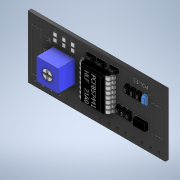
# Autodesk Inventor part: Part2_I2C
Saved by Autodesk Inventor 2021 (Build 250183000, 183)
## iProperties
Created: 2022-06-25
Part Number: Part2_I2C
Material: Generic
Document SubType Name: Modeling
Designer: Sam14
Density: 1 g/cm^3
Appearance: Chrome - Polished
Author: Sam14
Autodesk Inventor part; units mm, degrees
(part 1 of 3)
ref_plane "YZ Plane" through (0, 0, 0) normal (1, 0, 0) x (0, 1, 0)
ref_plane "XZ Plane" through (0, 0, 0) normal (0, 1, 0) x (-1, 0, 0)
sketch "Sketch1" plane through (0, 0, 0) normal (0, 0, 1) x (1, 0, 0)
  line L0 (0, 0) -> (38.1, 0)
  line L1 (0.325, -0.325) -> (0.325, 0.325)
  line L2 (0.325, 0.325) -> (-0.325, 0.325)
  line L3 (-0.325, 0.325) -> (-0.325, -0.325)
  line L4 (-0.325, -0.325) -> (0.325, -0.325)
  line L5 (0.325, -0.325) -> (-0.325, 0.325) construction
  line L6 (0.325, 0.325) -> (-0.325, -0.325) construction
  line L7 (38.425, -0.325) -> (37.775, -0.325)
  line L8 (37.775, -0.325) -> (37.775, 0.325)
  line L9 (37.775, 0.325) -> (38.425, 0.325)
  line L10 (38.425, 0.325) -> (38.425, -0.325)
  line L11 (38.425, -0.325) -> (37.775, 0.325) construction
  line L12 (37.775, -0.325) -> (38.425, 0.325) construction
  line L13 (0, 0) -> (2.54, 0)
  line L14 (2.54, 0) -> (5.08, 0)
  line L15 (5.08, 0) -> (7.62, 0)
  line L16 (7.62, 0) -> (10.16, 0)
  line L17 (10.16, 0) -> (12.7, 0)
  line L18 (12.7, 0) -> (15.24, 0)
  line L19 (15.24, 0) -> (17.78, 0)
  line L20 (17.78, 0) -> (20.32, 0)
  line L21 (20.32, 0) -> (22.86, 0)
  line L22 (22.86, 0) -> (25.4, 0)
  line L23 (25.4, 0) -> (27.94, 0)
  line L24 (27.94, 0) -> (30.48, 0)
  line L25 (30.48, 0) -> (33.02, 0)
  line L26 (33.02, 0) -> (35.56, 0)
  line L27 (35.56, 0) -> (38.1, 0)
  line L28 (-0.325, 0.325) -> (0.325, -0.325)
  line L29 (0.325, 0.325) -> (-0.325, -0.325)
  line L30 (2.865, -0.325) -> (2.865, 0.325)
  line L31 (2.865, 0.325) -> (2.215, 0.325)
  line L32 (2.215, 0.325) -> (2.215, -0.325)
  line L33 (2.215, -0.325) -> (2.865, -0.325)
  line L34 (2.865, -0.325) -> (2.215, 0.325) construction
  line L35 (2.865, 0.325) -> (2.215, -0.325) construction
  line L36 (5.405, -0.325) -> (5.405, 0.325)
  line L37 (5.405, 0.325) -> (4.755, 0.325)
  line L38 (4.755, 0.325) -> (4.755, -0.325)
  line L39 (4.755, -0.325) -> (5.405, -0.325)
  line L40 (5.405, -0.325) -> (4.755, 0.325) construction
  line L41 (5.405, 0.325) -> (4.755, -0.325) construction
  line L42 (7.945, -0.325) -> (7.945, 0.325)
  line L43 (7.945, 0.325) -> (7.295, 0.325)
  line L44 (7.295, 0.325) -> (7.295, -0.325)
  line L45 (7.295, -0.325) -> (7.945, -0.325)
  line L46 (7.945, -0.325) -> (7.295, 0.325) construction
  line L47 (7.945, 0.325) -> (7.295, -0.325) construction
  line L48 (10.485, -0.325) -> (10.485, 0.325)
  line L49 (10.485, 0.325) -> (9.835, 0.325)
  line L50 (9.835, 0.325) -> (9.835, -0.325)
  line L51 (9.835, -0.325) -> (10.485, -0.325)
  line L52 (10.485, -0.325) -> (9.835, 0.325) construction
  line L53 (10.485, 0.325) -> (9.835, -0.325) construction
  line L54 (13.025, -0.325) -> (13.025, 0.325)
  line L55 (13.025, 0.325) -> (12.375, 0.325)
  line L56 (12.375, 0.325) -> (12.375, -0.325)
  line L57 (12.375, -0.325) -> (13.025, -0.325)
  line L58 (13.025, -0.325) -> (12.375, 0.325) construction
  line L59 (13.025, 0.325) -> (12.375, -0.325) construction
  line L60 (15.565, -0.325) -> (15.565, 0.325)
  line L61 (15.565, 0.325) -> (14.915, 0.325)
  line L62 (14.915, 0.325) -> (14.915, -0.325)
  line L63 (14.915, -0.325) -> (15.565, -0.325)
  line L64 (15.565, -0.325) -> (14.915, 0.325) construction
  line L65 (15.565, 0.325) -> (14.915, -0.325) construction
  line L66 (18.105, -0.325) -> (18.105, 0.325)
  line L67 (18.105, 0.325) -> (17.455, 0.325)
  line L68 (17.455, 0.325) -> (17.455, -0.325)
  line L69 (17.455, -0.325) -> (18.105, -0.325)
  line L70 (18.105, -0.325) -> (17.455, 0.325) construction
  line L71 (18.105, 0.325) -> (17.455, -0.325) construction
  line L72 (20.645, -0.325) -> (20.645, 0.325)
  line L73 (20.645, 0.325) -> (19.995, 0.325)
  line L74 (19.995, 0.325) -> (19.995, -0.325)
  line L75 (19.995, -0.325) -> (20.645, -0.325)
  line L76 (20.645, -0.325) -> (19.995, 0.325) construction
  line L77 (20.645, 0.325) -> (19.995, -0.325) construction
  line L78 (23.185, -0.325) -> (23.185, 0.325)
  line L79 (23.185, 0.325) -> (22.535, 0.325)
  line L80 (22.535, 0.325) -> (22.535, -0.325)
  line L81 (22.535, -0.325) -> (23.185, -0.325)
  line L82 (23.185, -0.325) -> (22.535, 0.325) construction
  line L83 (23.185, 0.325) -> (22.535, -0.325) construction
  line L84 (25.725, -0.325) -> (25.725, 0.325)
  line L85 (25.725, 0.325) -> (25.075, 0.325)
  line L86 (25.075, 0.325) -> (25.075, -0.325)
  line L87 (25.075, -0.325) -> (25.725, -0.325)
  line L88 (25.725, -0.325) -> (25.075, 0.325) construction
  line L89 (25.725, 0.325) -> (25.075, -0.325) construction
  line L90 (28.265, -0.325) -> (28.265, 0.325)
  line L91 (28.265, 0.325) -> (27.615, 0.325)
  line L92 (27.615, 0.325) -> (27.615, -0.325)
  line L93 (27.615, -0.325) -> (28.265, -0.325)
  line L94 (28.265, -0.325) -> (27.615, 0.325) construction
  line L95 (28.265, 0.325) -> (27.615, -0.325) construction
  line L96 (30.805, -0.325) -> (30.805, 0.325)
  line L97 (30.805, 0.325) -> (30.155, 0.325)
  line L98 (30.155, 0.325) -> (30.155, -0.325)
  line L99 (30.155, -0.325) -> (30.805, -0.325)
  line L100 (30.805, -0.325) -> (30.155, 0.325) construction
  line L101 (30.805, 0.325) -> (30.155, -0.325) construction
  line L102 (33.345, -0.325) -> (33.345, 0.325)
  line L103 (33.345, 0.325) -> (32.695, 0.325)
  line L104 (32.695, 0.325) -> (32.695, -0.325)
  line L105 (32.695, -0.325) -> (33.345, -0.325)
  line L106 (33.345, -0.325) -> (32.695, 0.325) construction
  line L107 (33.345, 0.325) -> (32.695, -0.325) construction
  line L108 (35.885, -0.325) -> (35.885, 0.325)
  line L109 (35.885, 0.325) -> (35.235, 0.325)
  line L110 (35.235, 0.325) -> (35.235, -0.325)
  line L111 (35.235, -0.325) -> (35.885, -0.325)
  line L112 (35.885, -0.325) -> (35.235, 0.325) construction
  line L113 (35.885, 0.325) -> (35.235, -0.325) construction
  line L114 (0, 0) -> (-1.95, 0)
  line L115 (38.1, 0) -> (40.05, 0)
  line L116 (40.05, 0) -> (40.05, -1.5)
  line L117 (-1.95, 0) -> (-1.95, -1.5)
  line L118 (-1.95, -1.5) -> (40.05, -1.5)
  line L119 (40.05, -1.5) -> (40.05, 17.5)
  line L120 (-1.95, -1.5) -> (-1.95, 17.5)
  line L121 (-1.95, 17.5) -> (40.05, 17.5)
  dimension "d53" = 38.1
  dimension "d54" = 0.65
  dimension "d55" = 0.65
  dimension "d56" = 0.65
  dimension "d57" = 0.65
  dimension "d58" = 2.54
  dimension "d59" = 2.54
  dimension "d60" = 2.54
  dimension "d61" = 2.54
  dimension "d62" = 2.54
  dimension "d63" = 2.54
  dimension "d64" = 2.54
  dimension "d65" = 2.54
  dimension "d66" = 2.54
  dimension "d67" = 2.54
  dimension "d68" = 2.54
  dimension "d69" = 2.54
  dimension "d70" = 2.54
  dimension "d71" = 2.54
  dimension "d72" = 0.65
  dimension "d73" = 0.65
  dimension "d74" = 0.65
  dimension "d75" = 0.65
  dimension "d76" = 0.65
  dimension "d77" = 0.65
  dimension "d78" = 0.65
  dimension "d79" = 0.65
  dimension "d80" = 0.65
  dimension "d81" = 0.65
  dimension "d82" = 0.65
  dimension "d83" = 0.65
  dimension "d84" = 0.65
  dimension "d85" = 0.65
  dimension "d86" = 0.65
  dimension "d87" = 0.65
  dimension "d88" = 0.65
  dimension "d89" = 0.65
  dimension "d90" = 0.65
  dimension "d91" = 0.65
  dimension "d92" = 0.65
  dimension "d93" = 0.65
  dimension "d94" = 0.65
  dimension "d95" = 0.65
  dimension "d96" = 0.65
  dimension "d97" = 0.65
  dimension "d98" = 0.65
  dimension "d99" = 0.65
  dimension "d100" = 1.95
  dimension "d101" = 1.95
  dimension "d102" = 1.5
  dimension "d103" = 1.5
  dimension "d104" = 19
  dimension "d105" = 19
  constraints: 242 end point, 32 parallel, 18 vertical, 16 perpendicular, 4 midpoint, 3 horizontal, 1 point on line, 17 other
  measures "d53" distance of L13.start L27.end
  measures "d54" distance of L1.start L1.end
  measures "d55" distance of L2.end L1.end
  measures "d56" distance of L7.start L7.end
  measures "d57" distance of L7.end L8.end
  measures "d58" distance of L13.start L13.end
  measures "d59" distance of L13.end L14.end
  measures "d60" distance of L14.end L15.end
  measures "d61" distance of L15.end L16.end
  measures "d62" distance of L16.end L17.end
  measures "d63" distance of L17.end L18.end
  measures "d64" distance of L18.end L19.end
  measures "d65" distance of L19.end L20.end
  measures "d66" distance of L20.end L21.end
  measures "d67" distance of L21.end L22.end
  measures "d68" distance of L22.end L23.end
  measures "d69" distance of L23.end L24.end
  measures "d70" distance of L24.end L25.end
  measures "d71" distance of L25.end L26.end
  measures "d72" distance of L34.start L31.start
  measures "d73" distance of L31.end L31.start
  measures "d74" distance of L40.start L37.start
  measures "d75" distance of L37.end L37.start
  measures "d76" distance of L46.start L43.start
  measures "d77" distance of L43.end L43.start
  measures "d78" distance of L52.start L49.start
  measures "d79" distance of L49.end L49.start
  measures "d80" distance of L58.start L55.start
  measures "d81" distance of L55.end L55.start
  measures "d82" distance of L64.start L61.start
  measures "d83" distance of L61.end L61.start
  measures "d84" distance of L70.start L67.start
  measures "d85" distance of L67.end L67.start
  measures "d86" distance of L76.start L73.start
  measures "d87" distance of L73.end L73.start
  measures "d88" distance of L82.start L79.start
  measures "d89" distance of L79.end L79.start
  measures "d90" distance of L88.start L85.start
  measures "d91" distance of L85.end L85.start
  measures "d92" distance of L94.start L91.start
  measures "d93" distance of L91.end L91.start
  measures "d94" distance of L100.start L97.start
  measures "d95" distance of L97.end L97.start
  measures "d96" distance of L106.start L103.start
  measures "d97" distance of L103.end L103.start
  measures "d98" distance of L112.start L109.start
  measures "d99" distance of L109.end L109.start
  measures "d100" distance of L13.start L114.end
  measures "d101" distance of L27.end L115.end
  measures "d102" distance of L115.end L116.end
  measures "d103" distance of L114.end L117.end
  measures "d104" distance of L116.end L119.end
  measures "d105" distance of L117.end L120.end
extrude "Extrusion1" add sketch "Sketch1" along normal blind 1 contours L1 L2 L3 L114 L120 L121 L119 L115 L10 L9 L8 L0 L108 L109 L110 L102 L103 L104 L96 L97 L98 L90 L91 L92 L84 L85 L86 L78 L79 L80 L72 L73 L74 L66 L67 L68 L60 L61 L62 L54 L55 L56 L48 L49 L50 L42 L43 L44 L36 L37 L38 L30 L31 L32 | L0 L32 L33 L30 L38 L39 L36 L44 L45 L42 L50 L51 L48 L56 L57 L54 L62 L63 L60 L68 L69 L66 L74 L75 L72 L80 L81 L78 L86 L87 L84 L92 L93 L90 L98 L99 L96 L104 L105 L102 L110 L111 L108 L8 L7 L10 L115 L116 L118 L117 L114 L3 L4 L1
sketch "Sketch2" plane through (0, 0, 1) normal (0, 0, 1) x (1, 0, 0)
  line L0 (5.55, 12) -> (12.55, 12)
  line L1 (12.55, 12) -> (12.55, 5)
  line L2 (12.55, 5) -> (5.55, 5)
  line L3 (5.55, 5) -> (5.55, 12)
  line L4 (5.65, 5.1) -> (12.45, 5.1)
  line L5 (12.45, 5.1) -> (12.45, 11.9)
  line L6 (12.45, 11.9) -> (5.65, 11.9)
  line L7 (5.65, 11.9) -> (5.65, 5.1)
  line L8 (-0.95, 14.5) -> (-0.95, 1.5)
  line L9 (2.05, 14.5) -> (2.05, 1.5)
  line L10 (-0.95, 14.5) -> (2.05, 14.5)
  line L11 (-0.95, 1.5) -> (2.05, 1.5)
  line L12 (1.95, 14.4) -> (1.95, 1.6)
  line L13 (1.95, 1.6) -> (-0.85, 1.6)
  line L14 (-0.85, 1.6) -> (-0.85, 14.4)
  line L15 (-0.85, 14.4) -> (1.95, 14.4)
  line L16 (40.05, -1.5) -> (40.05, 17.5) projected
  line L17 (36.05, 4) -> (36.05, 12)
  line L18 (36.05, 12) -> (39.05, 12)
  line L19 (39.05, 4) -> (36.05, 4)
  line L20 (39.05, 12) -> (39.05, 4)
  line L21 (39.15, 12.1) -> (35.95, 12.1)
  line L22 (35.95, 12.1) -> (35.95, 3.9)
  line L23 (35.95, 3.9) -> (39.15, 3.9)
  line L24 (39.15, 3.9) -> (39.15, 12.1)
  line L25 (34.95, 3.9) -> (34.95, 6.4)
  line L26 (34.95, 6.4) -> (30.95, 6.4)
  line L27 (30.95, 6.4) -> (30.95, 3.9)
  line L28 (30.95, 3.9) -> (34.95, 3.9)
  line L29 (34.85, 4) -> (34.85, 6.3)
  line L30 (34.85, 6.3) -> (31.05, 6.3)
  line L31 (31.05, 6.3) -> (31.05, 4)
  line L32 (31.05, 4) -> (34.85, 4)
  line L33 (29.95, 3.9) -> (29.95, 6.9)
  line L34 (29.95, 6.9) -> (28.45, 6.9)
  line L35 (28.45, 6.9) -> (28.45, 3.9)
  line L36 (28.45, 3.9) -> (29.95, 3.9)
  line L37 (39.15, 3.9) -> (40.05, 3.9)
  line L38 (29.85, 6.8) -> (29.85, 4)
  line L39 (29.85, 4) -> (28.55, 4)
  line L40 (28.55, 4) -> (28.55, 6.8)
  line L41 (28.55, 6.8) -> (29.85, 6.8)
  line L42 (28.45, 3.9) -> (28.45, 6.9)
  line L43 (28.45, 6.9) -> (26.95, 6.9)
  line L44 (26.95, 6.9) -> (26.95, 3.9)
  line L45 (26.95, 3.9) -> (28.45, 3.9)
  line L46 (28.35, 6.8) -> (28.35, 4)
  line L47 (28.35, 4) -> (27.05, 4)
  line L48 (27.05, 4) -> (27.05, 6.8)
  line L49 (27.05, 6.8) -> (28.35, 6.8)
  line L50 (26.95, 3.9) -> (26.95, 6.9)
  line L51 (26.95, 6.9) -> (25.45, 6.9)
  line L52 (25.45, 6.9) -> (25.45, 3.9)
  line L53 (25.45, 3.9) -> (26.95, 3.9)
  line L54 (26.85, 6.8) -> (26.85, 4)
  line L55 (26.85, 4) -> (25.55, 4)
  line L56 (25.55, 4) -> (25.55, 6.8)
  line L57 (25.55, 6.8) -> (26.85, 6.8)
  line L58 (34.95, 10.5872) -> (34.95, 13.5872)
  line L59 (34.95, 13.5872) -> (33.45, 13.5872)
  line L60 (33.45, 13.5872) -> (33.45, 10.5872)
  line L61 (33.45, 10.5872) -> (34.95, 10.5872)
  line L62 (34.85, 13.4872) -> (34.85, 10.6872)
  line L63 (34.85, 10.6872) -> (33.55, 10.6872)
  line L64 (33.55, 10.6872) -> (33.55, 13.4872)
  line L65 (33.55, 13.4872) -> (34.85, 13.4872)
  line L66 (33.1382, 10.6872) -> (33.1382, 13.6872)
  line L67 (33.1382, 13.6872) -> (31.6382, 13.6872)
  line L68 (31.6382, 13.6872) -> (31.6382, 10.6872)
  line L69 (31.6382, 10.6872) -> (33.1382, 10.6872)
  line L70 (33.0382, 13.5872) -> (33.0382, 10.7872)
  line L71 (33.0382, 10.7872) -> (31.7382, 10.7872)
  line L72 (31.7382, 10.7872) -> (31.7382, 13.5872)
  line L73 (31.7382, 13.5872) -> (33.0382, 13.5872)
  line L74 (31.3887, 10.6872) -> (31.3887, 13.6872)
  line L75 (31.3887, 13.6872) -> (29.8887, 13.6872)
  line L76 (29.8887, 13.6872) -> (29.8887, 10.6872)
  line L77 (29.8887, 10.6872) -> (31.3887, 10.6872)
  line L78 (31.2887, 13.5872) -> (31.2887, 10.7872)
  line L79 (31.2887, 10.7872) -> (29.9887, 10.7872)
  line L80 (29.9887, 10.7872) -> (29.9887, 13.5872)
  line L81 (29.9887, 13.5872) -> (31.2887, 13.5872)
  line L82 (29.5585, 10.6872) -> (29.5585, 13.6872)
  line L83 (29.5585, 13.6872) -> (28.0585, 13.6872)
  line L84 (28.0585, 13.6872) -> (28.0585, 10.6872)
  line L85 (28.0585, 10.6872) -> (29.5585, 10.6872)
  line L86 (29.4585, 13.5872) -> (29.4585, 10.7872)
  line L87 (29.4585, 10.7872) -> (28.1585, 10.7872)
  line L88 (28.1585, 10.7872) -> (28.1585, 13.5872)
  line L89 (28.1585, 13.5872) -> (29.4585, 13.5872)
  line L90 (7.1408, 13.077) -> (7.1408, 16.077)
  line L91 (7.1408, 16.077) -> (5.6408, 16.077)
  line L92 (5.6408, 16.077) -> (5.6408, 13.077)
  line L93 (5.6408, 13.077) -> (7.1408, 13.077)
  line L94 (7.0408, 15.977) -> (7.0408, 13.177)
  line L95 (7.0408, 13.177) -> (5.7408, 13.177)
  line L96 (5.7408, 13.177) -> (5.7408, 15.977)
  line L97 (5.7408, 15.977) -> (7.0408, 15.977)
  line L98 (9.8434, 13.0715) -> (9.8434, 16.0715)
  line L99 (9.8434, 16.0715) -> (8.3434, 16.0715)
  line L100 (8.3434, 16.0715) -> (8.3434, 13.0715)
  line L101 (8.3434, 13.0715) -> (9.8434, 13.0715)
  line L102 (9.7434, 15.9715) -> (9.7434, 13.1715)
  line L103 (9.7434, 13.1715) -> (8.4434, 13.1715)
  line L104 (8.4434, 13.1715) -> (8.4434, 15.9715)
  line L105 (8.4434, 15.9715) -> (9.7434, 15.9715)
  line L106 (12.545, 13.0887) -> (12.545, 16.0887)
  line L107 (12.545, 16.0887) -> (11.045, 16.0887)
  line L108 (11.045, 16.0887) -> (11.045, 13.0887)
  line L109 (11.045, 13.0887) -> (12.545, 13.0887)
  line L110 (12.445, 15.9887) -> (12.445, 13.1887)
  line L111 (12.445, 13.1887) -> (11.145, 13.1887)
  line L112 (11.145, 13.1887) -> (11.145, 15.9887)
  line L113 (11.145, 15.9887) -> (12.445, 15.9887)
  line L114 (-1.95, 17.5) -> (-1.95, -1.5) projected
  line L115 (-1.95, 17.5) -> (16.05, 17.5)
  line L116 (40.05, 17.5) -> (-1.95, 17.5) projected
  line L117 (16.05, 14) -> (23.45, 14)
  line L118 (23.45, 14) -> (23.45, 3.5)
  line L119 (23.45, 3.5) -> (16.05, 3.5)
  line L120 (16.05, 3.5) -> (16.05, 14)
  line L121 (15.95, 14.1) -> (23.55, 14.1)
  line L122 (23.55, 14.1) -> (23.55, 3.4)
  line L123 (23.55, 3.4) -> (15.95, 3.4)
  line L124 (15.95, 3.4) -> (15.95, 14.1)
  line L125 (19.0957, 15.9376) -> (16.0957, 15.9376)
  line L126 (16.1957, 15.8376) -> (18.9957, 15.8376)
  line L127 (18.9957, 15.8376) -> (18.9957, 14.5376)
  line L128 (19.0957, 14.4376) -> (19.0957, 15.9376)
  line L129 (18.9957, 14.5376) -> (16.1957, 14.5376)
  line L130 (16.1957, 14.5376) -> (16.1957, 15.8376)
  line L131 (16.0957, 14.4376) -> (19.0957, 14.4376)
  line L132 (16.0957, 15.9376) -> (16.0957, 14.4376)
  line L133 (22.1559, 15.8398) -> (22.1559, 14.5398)
  line L134 (19.2559, 15.9398) -> (19.2559, 14.4398)
  line L135 (19.2559, 14.4398) -> (22.2559, 14.4398)
  line L136 (22.2559, 14.4398) -> (22.2559, 15.9398)
  line L137 (19.3559, 14.5398) -> (19.3559, 15.8398)
  line L138 (19.3559, 15.8398) -> (22.1559, 15.8398)
  line L139 (22.1559, 14.5398) -> (19.3559, 14.5398)
  line L140 (22.2559, 15.9398) -> (19.2559, 15.9398)
  line L141 (26.0246, 15.977) -> (26.0246, 14.677)
  line L142 (23.1246, 16.077) -> (23.1246, 14.577)
  line L143 (23.1246, 14.577) -> (26.1246, 14.577)
  line L144 (26.1246, 14.577) -> (26.1246, 16.077)
  line L145 (23.2246, 14.677) -> (23.2246, 15.977)
  line L146 (23.2246, 15.977) -> (26.0246, 15.977)
  line L147 (26.0246, 14.677) -> (23.2246, 14.677)
  line L148 (26.1246, 16.077) -> (23.1246, 16.077)
  point P0 (0, 0)
  dimension "d111" = 7
  dimension "d112" = 0.1
  dimension "d114" = 3
  dimension "d117" = 0.1
  dimension "d121" = 0.1
  dimension "d123" = 2.5
  dimension "d124" = 4
  dimension "d125" = 0.1
  dimension "d126" = 1
  dimension "d127" = 3
  dimension "d128" = 1.5
  dimension "d129" = 0.9
  dimension "d131" = 0.1
  dimension "d132" = 3
  dimension "d133" = 1.5
  dimension "d134" = 0.1
  dimension "d135" = 3
  dimension "d136" = 1.5
  dimension "d137" = 0.1
  dimension "d138" = 3
  dimension "d139" = 1.5
  dimension "d140" = 0.1
  dimension "d141" = 3
  dimension "d142" = 1.5
  dimension "d143" = 0.1
  dimension "d144" = 3
  dimension "d145" = 1.5
  dimension "d146" = 0.1
  dimension "d147" = 3
  dimension "d148" = 1.5
  dimension "d149" = 0.1
  dimension "d150" = 3
  dimension "d151" = 1.5
  dimension "d152" = 0.1
  dimension "d153" = 3
  dimension "d154" = 1.5
  dimension "d155" = 0.1
  dimension "d156" = 3
  dimension "d157" = 1.5
  dimension "d158" = 0.1
  dimension "d159" = 18
  dimension "d160" = 3.5
  dimension "d161" = 7.4
  dimension "d162" = 10.5
  dimension "d163" = 0.1
  dimension "d164" = 3
  dimension "d165" = 1.5
  dimension "d166" = 0.1
  dimension "d167" = 3
  dimension "d168" = 1.5
  dimension "d169" = 0.1
  dimension "d170" = 3
  dimension "d171" = 1.5
  dimension "d172" = 0.1
  constraints: 292 end point, 100 perpendicular, 3 point on line, 2 parallel, 1 horizontal, 1 vertical, 54 other
  measures "d111" distance of L0.end L1.end
  measures "d112" distance between parallel lines of L2 L4
  measures "d114" distance between parallel lines of L8 L9
  measures "d117" distance between parallel lines of L10 L15
  measures "d121" distance between parallel lines of L18 L21
  measures "d123" distance of L25.start L25.end
  measures "d124" distance of L25.end L26.end
  measures "d125" distance between parallel lines of L28 L32
  measures "d126" distance of L27.end L33.start
  measures "d127" distance of L33.start L33.end
  measures "d128" distance of L33.end L34.end
  measures "d129" distance of L23.end L37.end
  measures "d131" distance between parallel lines of L33 L38
  measures "d132" distance of L42.start L43.start
  measures "d133" distance of L43.start L44.start
  measures "d134" distance between parallel lines of L42 L46
  measures "d135" distance of L50.start L51.start
  measures "d136" distance of L51.start L52.start
  measures "d137" distance between parallel lines of L50 L54
  measures "d138" distance of L58.start L59.start
  measures "d139" distance of L59.start L60.start
  measures "d140" distance between parallel lines of L58 L62
  measures "d141" distance of L66.start L67.start
  measures "d142" distance of L67.start L68.start
  measures "d143" distance between parallel lines of L66 L70
  measures "d144" distance of L74.start L75.start
  measures "d145" distance of L75.start L76.start
  measures "d146" distance between parallel lines of L74 L78
  measures "d147" distance of L82.start L83.start
  measures "d148" distance of L83.start L84.start
  measures "d149" distance between parallel lines of L82 L86
  measures "d150" distance of L90.start L91.start
  measures "d151" distance of L91.start L92.start
  measures "d152" distance between parallel lines of L90 L94
  measures "d153" distance of L98.start L99.start
  measures "d154" distance of L99.start L100.start
  measures "d155" distance between parallel lines of L98 L102
  measures "d156" distance of L106.start L107.start
  measures "d157" distance of L107.start L108.start
  measures "d158" distance between parallel lines of L106 L110
  measures "d159" distance of L114.start L115.end
  measures "d160" distance of L115.end L117.start
  measures "d161" distance of L117.start L117.end
  measures "d162" distance of L117.end L118.end
  measures "d163" distance between parallel lines of L120 L124
  measures "d164" distance of L132.end L131.end
  measures "d165" distance of L131.end L128.end
  measures "d166" distance between parallel lines of L131 L129
  measures "d167" distance of L134.end L136.start
  measures "d168" distance of L136.start L140.start
  measures "d169" distance between parallel lines of L135 L139
  measures "d170" distance of L142.end L144.start
  measures "d171" distance of L144.start L148.start
  measures "d172" distance between parallel lines of L143 L147
extrude "Extrusion2" add sketch "Sketch2" along normal blind 0.1
sketch "Sketch4" plane through (0, 0, 1) normal (0, 0, 1) x (1, 0, 0)
  line L0 (5.65, 5.1) -> (12.45, 5.1) projected
  line L1 (12.45, 5.1) -> (12.45, 11.9) projected
  line L2 (12.45, 11.9) -> (5.65, 11.9) projected
  line L3 (5.65, 11.9) -> (5.65, 5.1) projected
  line L4 (5.75, 11.8) -> (12.35, 11.8)
  line L5 (12.35, 11.8) -> (12.35, 5.2)
  line L6 (12.35, 5.2) -> (5.75, 5.2)
  line L7 (5.75, 5.2) -> (5.75, 11.8)
  point P0 (0, 0)
  dimension "d175" = 0.1
  constraints: 8 end point, 3 other
  measures "d175" distance between parallel lines of L2 L4
extrude "Extrusion3" add sketch "Sketch4" along normal blind 5.1 contours L4 L5 L6 L7
sketch "Sketch5" plane through (0, 0, 6.1) normal (0, 0, 1) x (1, 0, 0)
  line L0 (5.75, 5.2) -> (12.35, 5.2) projected
  line L1 (12.35, 5.2) -> (12.35, 11.8) projected
  line L2 (12.35, 11.8) -> (5.75, 11.8) projected
  line L3 (5.75, 11.8) -> (5.75, 5.2) projected
  line L4 (5.75, 11.8) -> (12.35, 5.2)
  line L5 (5.75, 5.2) -> (12.35, 11.8)
  circle A0 centre (9.05, 8.5) radius 1.5
  point P0 (0, 0)
  dimension "d178" = 3
  constraints: 4 end point, 1 centre point, 1 midpoint, 1 perpendicular
  measures "d178" diameter of A0
extrude "Extrusion4" cut sketch "Sketch5" against normal blind 1 contours A0 L4 L5 | L5 L4 A0 | L4 L5 A0 | A0 L5 L4
sketch "Sketch6" plane through (0, 0, 6.1) normal (0, 0, 1) x (1, 0, 0)
  circle A0 centre (9.05, 8.5) radius 1.5 projected
  circle A1 centre (9.05, 8.5) radius 1.75
  circle A2 centre (9.05, 8.5) radius 1.85
  point P0 (0, 0)
  dimension "d181" = 3.5
  dimension "d182" = 3.7
  constraints: 2 centre point, 2 coincident
  measures "d181" diameter of A1
  measures "d182" diameter of A2
extrude "Extrusion5" cut sketch "Sketch6" against normal blind 0.25 contours A2
sketch "Sketch7" plane through (9.05, 8.5, 5.1) normal (0, 0, 1) x (1, 0, 0)
  circle A0 centre (0, 0) radius 1.5 projected
  line L0 (0.25, -1.5) -> (0.25, 1.5)
  line L1 (0.25, 1.5) -> (-0.25, 1.5)
  line L2 (-0.25, 1.5) -> (-0.25, -1.5)
  line L3 (-0.25, -1.5) -> (0.25, -1.5)
  line L4 (0.25, -1.5) -> (-0.25, 1.5) construction
  line L5 (0.25, 1.5) -> (-0.25, -1.5) construction
  line L6 (-1.5, -0.25) -> (1.5, -0.25)
  line L7 (1.5, -0.25) -> (1.5, 0.25)
  line L8 (1.5, 0.25) -> (-1.5, 0.25)
  line L9 (-1.5, 0.25) -> (-1.5, -0.25)
  line L10 (-1.5, -0.25) -> (1.5, 0.25) construction
  line L11 (1.5, -0.25) -> (-1.5, 0.25) construction
  point P0 (-9.05, -8.5)
  point P1 (1.479, -0.25)
  point P2 (0.25, -0.25)
  point P3 (0.25, -1.479)
  point P4 (-0.25, -0.25)
  point P5 (-1.479, -0.25)
  point P6 (-0.25, -1.479)
  point P7 (0.25, 0.25)
  point P8 (1.479, 0.25)
  point P9 (0.25, 1.479)
  point P10 (-1.479, 0.25)
  point P11 (-0.25, 0.25)
  point P12 (-0.25, 1.479)
  dimension "d185" = 0.5
  dimension "d186" = 0.5
  constraints: 24 end point, 4 midpoint, 4 parallel, 2 perpendicular, 1 horizontal, 1 vertical
  measures "d185" distance of L1.end L0.end
  measures "d186" distance of L7.end L6.end
extrude "Extrusion6" add sketch "Sketch7" along normal blind 1.01 contours L8 L0 A0 | A0 L0 L6 | L8 A0 L2 | L2 A0 L6
sketch "Sketch8" plane through (0, 0, 1) normal (0, 0, 1) x (1, 0, 0)
  line L0 (8.3434, 13.0715) -> (8.3434, 16.0715) projected
  line L1 (8.3434, 16.0715) -> (9.8434, 16.0715) projected
  line L2 (9.8434, 16.0715) -> (9.8434, 13.0715) projected
  line L3 (9.8434, 13.0715) -> (8.3434, 13.0715) projected
  line L4 (19.2559, 14.4398) -> (19.2559, 15.9398) projected
  line L5 (19.2559, 15.9398) -> (22.2559, 15.9398) projected
  line L6 (22.2559, 15.9398) -> (22.2559, 14.4398) projected
  line L7 (22.2559, 14.4398) -> (19.2559, 14.4398) projected
  line L8 (29.8887, 10.6872) -> (29.8887, 13.6872) projected
  line L9 (29.8887, 13.6872) -> (31.3887, 13.6872) projected
  line L10 (31.3887, 13.6872) -> (31.3887, 10.6872) projected
  line L11 (31.3887, 10.6872) -> (29.8887, 10.6872) projected
  line L12 (34.95, 6.4) -> (34.95, 3.9) projected
  line L13 (34.95, 3.9) -> (30.95, 3.9) projected
  line L14 (30.95, 3.9) -> (30.95, 6.4) projected
  line L15 (30.95, 6.4) -> (34.95, 6.4) projected
  line L16 (25.45, 6.9) -> (29.95, 6.9) projected
  line L17 (29.95, 6.9) -> (29.95, 3.9) projected
  line L18 (29.95, 3.9) -> (25.45, 3.9) projected
  line L19 (25.45, 3.9) -> (25.45, 6.9) projected
  line L20 (28.0585, 10.6872) -> (28.0585, 13.6872) projected
  line L21 (28.0585, 13.6872) -> (29.5585, 13.6872) projected
  line L22 (29.5585, 13.6872) -> (29.5585, 10.6872) projected
  line L23 (29.5585, 10.6872) -> (28.0585, 10.6872) projected
  line L24 (16.0957, 14.4376) -> (16.0957, 15.9376) projected
  line L25 (16.0957, 15.9376) -> (19.0957, 15.9376) projected
  line L26 (19.0957, 15.9376) -> (19.0957, 14.4376) projected
  line L27 (19.0957, 14.4376) -> (16.0957, 14.4376) projected
  line L28 (5.6408, 13.077) -> (5.6408, 16.077) projected
  line L29 (5.6408, 16.077) -> (7.1408, 16.077) projected
  line L30 (7.1408, 16.077) -> (7.1408, 13.077) projected
  line L31 (7.1408, 13.077) -> (5.6408, 13.077) projected
  line L32 (11.045, 13.0887) -> (11.045, 16.0887) projected
  line L33 (11.045, 16.0887) -> (12.545, 16.0887) projected
  line L34 (12.545, 16.0887) -> (12.545, 13.0887) projected
  line L35 (12.545, 13.0887) -> (11.045, 13.0887) projected
  line L36 (23.1246, 14.577) -> (23.1246, 16.077) projected
  line L37 (23.1246, 16.077) -> (26.1246, 16.077) projected
  line L38 (26.1246, 16.077) -> (26.1246, 14.577) projected
  line L39 (26.1246, 14.577) -> (23.1246, 14.577) projected
  line L40 (31.6382, 10.6872) -> (31.6382, 13.6872) projected
  line L41 (31.6382, 13.6872) -> (33.1382, 13.6872) projected
  line L42 (33.1382, 13.6872) -> (33.1382, 10.6872) projected
  line L43 (33.1382, 10.6872) -> (31.6382, 10.6872) projected
  line L44 (39.15, 12.1) -> (39.15, 3.9) projected
  line L45 (39.15, 3.9) -> (35.95, 3.9) projected
  line L46 (35.95, 3.9) -> (35.95, 12.1) projected
  line L47 (35.95, 12.1) -> (39.15, 12.1) projected
  line L48 (33.45, 10.5872) -> (33.45, 13.5872) projected
  line L49 (33.45, 13.5872) -> (34.95, 13.5872) projected
  line L50 (34.95, 13.5872) -> (34.95, 10.5872) projected
  line L51 (34.95, 10.5872) -> (33.45, 10.5872) projected
  line L52 (15.95, 3.4) -> (15.95, 14.1) projected
  line L53 (15.95, 14.1) -> (23.55, 14.1) projected
  line L54 (23.55, 14.1) -> (23.55, 3.4) projected
  line L55 (23.55, 3.4) -> (15.95, 3.4) projected
  line L56 (5.55, 5) -> (5.55, 12) projected
  line L57 (5.55, 12) -> (12.55, 12) projected
  line L58 (12.55, 12) -> (12.55, 5) projected
  line L59 (12.55, 5) -> (5.55, 5) projected
  line L60 (-0.95, 14.5) -> (2.05, 14.5) projected
  line L61 (2.05, 14.5) -> (2.05, 1.5) projected
  line L62 (2.05, 1.5) -> (-0.95, 1.5) projected
  line L63 (-0.95, 1.5) -> (-0.95, 14.5) projected
  line L64 (40.05, 17.5) -> (-1.95, 17.5) projected
  line L65 (-1.95, 17.5) -> (-1.95, -1.5) projected
  line L66 (-1.95, -1.5) -> (40.05, -1.5) projected
  line L67 (40.05, -1.5) -> (40.05, 17.5) projected
  line L68 (2.215, -0.325) -> (2.215, 0.325) projected
  line L69 (2.215, 0.325) -> (2.865, 0.325) projected
  line L70 (2.865, 0.325) -> (2.865, -0.325) projected
  line L71 (2.865, -0.325) -> (2.215, -0.325) projected
  line L72 (4.755, -0.325) -> (4.755, 0.325) projected
  line L73 (4.755, 0.325) -> (5.405, 0.325) projected
  line L74 (5.405, 0.325) -> (5.405, -0.325) projected
  line L75 (5.405, -0.325) -> (4.755, -0.325) projected
  line L76 (7.295, -0.325) -> (7.295, 0.325) projected
  line L77 (7.295, 0.325) -> (7.945, 0.325) projected
  line L78 (7.945, 0.325) -> (7.945, -0.325) projected
  line L79 (7.945, -0.325) -> (7.295, -0.325) projected
  line L80 (9.835, -0.325) -> (9.835, 0.325) projected
  line L81 (9.835, 0.325) -> (10.485, 0.325) projected
  line L82 (10.485, 0.325) -> (10.485, -0.325) projected
  line L83 (10.485, -0.325) -> (9.835, -0.325) projected
  line L84 (12.375, -0.325) -> (12.375, 0.325) projected
  line L85 (12.375, 0.325) -> (13.025, 0.325) projected
  line L86 (13.025, 0.325) -> (13.025, -0.325) projected
  line L87 (13.025, -0.325) -> (12.375, -0.325) projected
  line L88 (14.915, -0.325) -> (14.915, 0.325) projected
  line L89 (14.915, 0.325) -> (15.565, 0.325) projected
  line L90 (15.565, 0.325) -> (15.565, -0.325) projected
  line L91 (15.565, -0.325) -> (14.915, -0.325) projected
  line L92 (17.455, -0.325) -> (17.455, 0.325) projected
  line L93 (17.455, 0.325) -> (18.105, 0.325) projected
  line L94 (18.105, 0.325) -> (18.105, -0.325) projected
  line L95 (18.105, -0.325) -> (17.455, -0.325) projected
  line L96 (19.995, -0.325) -> (19.995, 0.325) projected
  line L97 (19.995, 0.325) -> (20.645, 0.325) projected
  line L98 (20.645, 0.325) -> (20.645, -0.325) projected
  line L99 (20.645, -0.325) -> (19.995, -0.325) projected
  line L100 (22.535, -0.325) -> (22.535, 0.325) projected
  line L101 (22.535, 0.325) -> (23.185, 0.325) projected
  line L102 (23.185, 0.325) -> (23.185, -0.325) projected
  line L103 (23.185, -0.325) -> (22.535, -0.325) projected
  line L104 (25.075, -0.325) -> (25.075, 0.325) projected
  line L105 (25.075, 0.325) -> (25.725, 0.325) projected
  line L106 (25.725, 0.325) -> (25.725, -0.325) projected
  line L107 (25.725, -0.325) -> (25.075, -0.325) projected
  line L108 (27.615, -0.325) -> (27.615, 0.325) projected
  line L109 (27.615, 0.325) -> (28.265, 0.325) projected
  line L110 (28.265, 0.325) -> (28.265, -0.325) projected
  line L111 (28.265, -0.325) -> (27.615, -0.325) projected
  line L112 (30.155, -0.325) -> (30.155, 0.325) projected
  line L113 (30.155, 0.325) -> (30.805, 0.325) projected
  line L114 (30.805, 0.325) -> (30.805, -0.325) projected
  line L115 (30.805, -0.325) -> (30.155, -0.325) projected
  line L116 (32.695, -0.325) -> (32.695, 0.325) projected
  line L117 (32.695, 0.325) -> (33.345, 0.325) projected
  line L118 (33.345, 0.325) -> (33.345, -0.325) projected
  line L119 (33.345, -0.325) -> (32.695, -0.325) projected
  line L120 (35.235, -0.325) -> (35.235, 0.325) projected
  line L121 (35.235, 0.325) -> (35.885, 0.325) projected
  line L122 (35.885, 0.325) -> (35.885, -0.325) projected
  line L123 (35.885, -0.325) -> (35.235, -0.325) projected
  line L124 (37.775, -0.325) -> (37.775, 0.325) projected
  line L125 (37.775, 0.325) -> (38.425, 0.325) projected
  line L126 (38.425, 0.325) -> (38.425, -0.325) projected
  line L127 (38.425, -0.325) -> (37.775, -0.325) projected
  line L128 (0.325, 0.325) -> (0.325, -0.325) projected
  line L129 (0.325, -0.325) -> (-0.325, -0.325) projected
  line L130 (-0.325, -0.325) -> (-0.325, 0.325) projected
  line L131 (-0.325, 0.325) -> (0.325, 0.325) projected
  line L132 (11.145, 13.1887) -> (12.445, 13.1887) projected
  line L133 (12.445, 13.1887) -> (12.445, 15.9887) projected
  line L134 (12.445, 15.9887) -> (11.145, 15.9887) projected
  line L135 (11.145, 15.9887) -> (11.145, 13.1887) projected
  line L136 (8.4434, 13.1715) -> (9.7434, 13.1715) projected
  line L137 (9.7434, 13.1715) -> (9.7434, 15.9715) projected
  line L138 (9.7434, 15.9715) -> (8.4434, 15.9715) projected
  line L139 (8.4434, 15.9715) -> (8.4434, 13.1715) projected
  line L140 (5.7408, 13.177) -> (7.0408, 13.177) projected
  line L141 (7.0408, 13.177) -> (7.0408, 15.977) projected
  line L142 (7.0408, 15.977) -> (5.7408, 15.977) projected
  line L143 (5.7408, 15.977) -> (5.7408, 13.177) projected
  line L144 (11.245, 15.8887) -> (12.345, 15.8887)
  line L145 (12.345, 15.8887) -> (12.345, 13.2887)
  line L146 (12.345, 13.2887) -> (11.245, 13.2887)
  line L147 (11.245, 13.2887) -> (11.245, 15.8887)
  line L148 (9.6434, 15.8715) -> (9.6434, 13.2715)
  line L149 (9.6434, 13.2715) -> (8.5434, 13.2715)
  line L150 (8.5434, 13.2715) -> (8.5434, 15.8715)
  line L151 (8.5434, 15.8715) -> (9.6434, 15.8715)
  line L152 (6.9408, 15.877) -> (6.9408, 13.277)
  line L153 (6.9408, 13.277) -> (5.8408, 13.277)
  line L154 (5.8408, 13.277) -> (5.8408, 15.877)
  line L155 (5.8408, 15.877) -> (6.9408, 15.877)
  line L156 (6.9408, 14.577) -> (5.8408, 14.577)
  line L157 (6.9408, 14.377) -> (5.8408, 14.377)
  line L158 (6.9408, 14.777) -> (5.8408, 14.777)
  line L159 (9.6434, 14.377) -> (8.5434, 14.377)
  line L160 (9.6434, 14.777) -> (8.5434, 14.777)
  line L161 (12.345, 14.377) -> (11.245, 14.377)
  line L162 (12.345, 14.777) -> (11.245, 14.777)
  point P0 (0, 0)
  dimension "d189" = 0.1
  dimension "d190" = 0.1
  dimension "d191" = 0.1
  dimension "d192" = 0.2
  dimension "d193" = 0.2
  constraints: 38 end point, 2 midpoint, 2 parallel, 9 other
  measures "d189" distance between parallel lines of L134 L144
  measures "d190" distance between parallel lines of L137 L148
  measures "d191" distance between parallel lines of L141 L152
  measures "d192" distance between parallel lines of L156 L157
  measures "d193" distance between parallel lines of L156 L158
extrude "Extrusion7" add sketch "Sketch8" along normal blind 0.1 contours L144 L145 L162 L147 | L161 L145 L146 L147 | L148 L160 L150 L151 | L148 L149 L150 L159 | L152 L158 L154 L155 | L152 L153 L154 L157
sketch "Sketch9" plane through (0, 0, 1) normal (0, 0, 1) x (1, 0, 0)
  line L0 (26.0246, 14.677) -> (26.0246, 15.977) projected
  line L1 (26.0246, 15.977) -> (23.2246, 15.977) projected
  line L2 (23.2246, 15.977) -> (23.2246, 14.677) projected
  line L3 (23.2246, 14.677) -> (26.0246, 14.677) projected
  line L4 (22.1559, 14.5398) -> (22.1559, 15.8398) projected
  line L5 (22.1559, 15.8398) -> (19.3559, 15.8398) projected
  line L6 (19.3559, 15.8398) -> (19.3559, 14.5398) projected
  line L7 (19.3559, 14.5398) -> (22.1559, 14.5398) projected
  line L8 (18.9957, 15.8376) -> (16.1957, 15.8376) projected
  line L9 (16.1957, 15.8376) -> (16.1957, 14.5376) projected
  line L10 (16.1957, 14.5376) -> (18.9957, 14.5376) projected
  line L11 (18.9957, 14.5376) -> (18.9957, 15.8376) projected
  line L12 (18.8957, 15.7376) -> (16.2957, 15.7376)
  line L13 (16.2957, 15.7376) -> (16.2957, 14.6376)
  line L14 (16.2957, 14.6376) -> (18.8957, 14.6376)
  line L15 (18.8957, 14.6376) -> (18.8957, 15.7376)
  line L16 (19.4559, 14.6398) -> (19.4559, 15.7398)
  line L17 (19.4559, 15.7398) -> (22.0559, 15.7398)
  line L18 (22.0559, 15.7398) -> (22.0559, 14.6398)
  line L19 (22.0559, 14.6398) -> (19.4559, 14.6398)
  line L20 (23.3246, 14.777) -> (23.3246, 15.877)
  line L21 (23.3246, 15.877) -> (25.9246, 15.877)
  line L22 (25.9246, 15.877) -> (25.9246, 14.777)
  line L23 (25.9246, 14.777) -> (23.3246, 14.777)
  line L24 (25.55, 4) -> (26.85, 4) projected
  line L25 (26.85, 4) -> (26.85, 6.8) projected
  line L26 (26.85, 6.8) -> (25.55, 6.8) projected
  line L27 (25.55, 6.8) -> (25.55, 4) projected
  line L28 (27.05, 4) -> (28.35, 4) projected
  line L29 (28.35, 4) -> (28.35, 6.8) projected
  line L30 (28.35, 6.8) -> (27.05, 6.8) projected
  line L31 (27.05, 6.8) -> (27.05, 4) projected
  line L32 (29.85, 6.8) -> (28.55, 6.8) projected
  line L33 (28.55, 6.8) -> (28.55, 4) projected
  line L34 (28.55, 4) -> (29.85, 4) projected
  line L35 (29.85, 4) -> (29.85, 6.8) projected
  line L36 (28.1585, 10.7872) -> (29.4585, 10.7872) projected
  line L37 (29.4585, 10.7872) -> (29.4585, 13.5872) projected
  line L38 (29.4585, 13.5872) -> (28.1585, 13.5872) projected
  line L39 (28.1585, 13.5872) -> (28.1585, 10.7872) projected
  line L40 (29.9887, 10.7872) -> (31.2887, 10.7872) projected
  line L41 (31.2887, 10.7872) -> (31.2887, 13.5872) projected
  line L42 (31.2887, 13.5872) -> (29.9887, 13.5872) projected
  line L43 (29.9887, 13.5872) -> (29.9887, 10.7872) projected
  line L44 (31.7382, 10.7872) -> (33.0382, 10.7872) projected
  line L45 (33.0382, 10.7872) -> (33.0382, 13.5872) projected
  line L46 (33.0382, 13.5872) -> (31.7382, 13.5872) projected
  line L47 (31.7382, 13.5872) -> (31.7382, 10.7872) projected
  line L48 (33.55, 10.6872) -> (34.85, 10.6872) projected
  line L49 (34.85, 10.6872) -> (34.85, 13.4872) projected
  line L50 (34.85, 13.4872) -> (33.55, 13.4872) projected
  line L51 (33.55, 13.4872) -> (33.55, 10.6872) projected
  line L52 (34.85, 4) -> (34.85, 6.3) projected
  line L53 (34.85, 6.3) -> (31.05, 6.3) projected
  line L54 (31.05, 6.3) -> (31.05, 4) projected
  line L55 (31.05, 4) -> (34.85, 4) projected
  line L56 (26.95, 6.9) -> (26.95, 3.9)
  line L57 (26.95, 3.9) -> (25.45, 3.9)
  line L58 (25.45, 3.9) -> (25.45, 6.9)
  line L59 (25.45, 6.9) -> (26.95, 6.9)
  line L60 (27.15, 4.1) -> (28.25, 4.1)
  line L61 (28.25, 4.1) -> (28.25, 6.7)
  line L62 (28.25, 6.7) -> (27.15, 6.7)
  line L63 (27.15, 6.7) -> (27.15, 4.1)
  line L64 (25.65, 4.1) -> (26.75, 4.1)
  line L65 (26.75, 4.1) -> (26.75, 6.7)
  line L66 (26.75, 6.7) -> (25.65, 6.7)
  line L67 (25.65, 6.7) -> (25.65, 4.1)
  line L68 (28.65, 4.1) -> (28.65, 6.7)
  line L69 (28.65, 6.7) -> (29.75, 6.7)
  line L70 (29.75, 6.7) -> (29.75, 4.1)
  line L71 (29.75, 4.1) -> (28.65, 4.1)
  line L72 (34.75, 4.1) -> (34.75, 6.2)
  line L73 (34.75, 6.2) -> (31.15, 6.2)
  line L74 (31.15, 6.2) -> (31.15, 4.1)
  line L75 (31.15, 4.1) -> (34.75, 4.1)
  line L76 (33.65, 10.7872) -> (34.75, 10.7872)
  line L77 (34.75, 10.7872) -> (34.75, 13.3872)
  line L78 (34.75, 13.3872) -> (33.65, 13.3872)
  line L79 (33.65, 13.3872) -> (33.65, 10.7872)
  line L80 (32.9382, 13.4872) -> (32.9382, 10.8872)
  line L81 (32.9382, 10.8872) -> (31.8382, 10.8872)
  line L82 (31.8382, 10.8872) -> (31.8382, 13.4872)
  line L83 (31.8382, 13.4872) -> (32.9382, 13.4872)
  line L84 (31.1887, 13.4872) -> (31.1887, 10.8872)
  line L85 (31.1887, 10.8872) -> (30.0887, 10.8872)
  line L86 (30.0887, 10.8872) -> (30.0887, 13.4872)
  line L87 (30.0887, 13.4872) -> (31.1887, 13.4872)
  line L88 (29.3585, 13.4872) -> (29.3585, 10.8872)
  line L89 (29.3585, 10.8872) -> (28.2585, 10.8872)
  line L90 (28.2585, 10.8872) -> (28.2585, 13.4872)
  line L91 (28.2585, 13.4872) -> (29.3585, 13.4872)
  point P0 (0, 0)
  dimension "d196" = 0.1
  dimension "d197" = 0.1
  dimension "d198" = 0.1
  dimension "d199" = 0.1
  dimension "d200" = 0.1
  dimension "d201" = 0.1
  dimension "d202" = 0.1
  dimension "d203" = 0.1
  dimension "d204" = 0.1
  dimension "d205" = 0.1
  dimension "d206" = 0.1
  dimension "d207" = 0.1
  constraints: 96 end point, 36 other
  measures "d196" distance between parallel lines of L11 L15
  measures "d197" distance between parallel lines of L6 L16
  measures "d198" distance between parallel lines of L2 L20
  measures "d199" distance between parallel lines of L25 L56
  measures "d200" distance between parallel lines of L31 L63
  measures "d201" distance between parallel lines of L27 L67
  measures "d202" distance between parallel lines of L33 L68
  measures "d203" distance between parallel lines of L55 L75
  measures "d204" distance between parallel lines of L51 L79
  measures "d205" distance between parallel lines of L45 L80
  measures "d206" distance between parallel lines of L41 L84
  measures "d207" distance between parallel lines of L37 L88
extrude "Extrusion8" add sketch "Sketch9" along normal blind 1 contours L15 L14 L13 L12 | L16 L17 L18 L19 | L20 L21 L22 L23 | L63 L62 L61 L60 | L67 L66 L65 L64 | L68 L69 L70 L71 | L75 L74 L73 L72 | L79 L78 L77 L76 | L80 L81 L82 L83 | L84 L85 L86 L87 | L88 L89 L90 L91
chamfer "Chamfer1" distance 0.5 angle 45 20 edges at (16.2957, 15.1876, 2) (19.4559, 15.1898, 2) (18.8957, 15.1876, 2) (22.0559, 15.1898, 2) (23.3246, 15.327, 2) (25.9246, 15.327, 2) (32.3882, 10.8872, 2) (32.3882, 13.4872, 2) (30.6387, 13.4872, 2) (30.6387, 10.8872, 2) (28.8085, 10.8872, 2) (28.8085, 13.4872, 2) (29.2, 4.1, 2) (29.2, 6.7, 2) (27.7, 4.1, 2) (27.7, 6.7, 2) (26.2, 4.1, 2) (26.2, 6.7, 2) (34.2, 10.7872, 2) (34.2, 13.3872, 2)
sketch "Sketch10" plane through (0, 0, 1) normal (0, 0, 1) x (1, 0, 0)
  line L0 (16.05, 14) -> (16.05, 3.5) projected
  line L1 (16.05, 3.5) -> (23.45, 3.5) projected
  line L2 (23.45, 3.5) -> (23.45, 14) projected
  line L3 (23.45, 14) -> (16.05, 14) projected
  line L4 (16.15, 13.9) -> (16.15, 3.6)
  line L5 (16.15, 3.6) -> (23.35, 3.6)
  line L6 (23.35, 3.6) -> (23.35, 13.9)
  line L7 (23.35, 13.9) -> (16.15, 13.9)
  point P0 (0, 0)
  dimension "d213" = 0.1
  constraints: 8 end point, 3 other
  measures "d213" distance between parallel lines of L3 L7
extrude "Extrusion9" add sketch "Sketch10" along normal blind 2.5 contours L7 L6 L5 L4
chamfer "Chamfer2" distance 0.5 angle 45 4 edges at (16.15, 8.75, 3.5) (23.35, 8.75, 3.5) (19.75, 3.6, 3.5) (19.75, 13.9, 3.5)